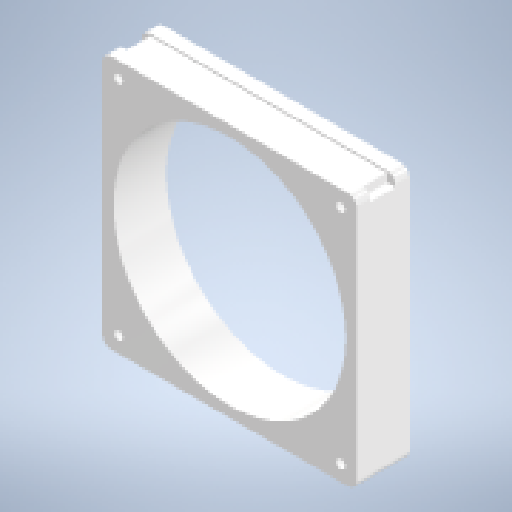
# Autodesk Inventor part: Body
Saved by Autodesk Inventor 2023.1 (Build 271208000, 208)
## iProperties
Created: 2023-11-19
Part Number: Body
Material: ABS Plastic
Document SubType Name: Modeling
Designer: Vinicius
Density: 1.06 g/cm^3
Appearance: Rubber - Black
Author: Vinicius
Autodesk Inventor part; units mm, degrees
ref_plane "YZ Plane" through (0, 0, 0) normal (1, 0, 0) x (0, 1, 0)
ref_plane "XZ Plane" through (0, 0, 0) normal (0, 1, 0) x (-1, 0, 0)
ref_plane "XY Plane" through (0, 0, 0) normal (0, 0, 1) x (1, 0, 0)
sketch "Sketch1" plane through (0, 0, 0) normal (0, 0, 1) x (1, 0, 0)
  line L0 (-56, 60) -> (56, 60)
  line L1 (60, 56) -> (60, -56)
  line L2 (56, -60) -> (-56, -60)
  line L3 (-60, -56) -> (-60, 56)
  line L4 (-60, 60) -> (60, -60) construction
  line L5 (60, 60) -> (-60, -60) construction
  circle A0 centre (0, 0) radius 55
  line L6 (-52.5, 52.5) -> (52.5, 52.5) construction
  line L7 (52.5, 52.5) -> (52.5, -52.5) construction
  line L8 (52.5, -52.5) -> (-52.5, -52.5) construction
  line L9 (-52.5, -52.5) -> (-52.5, 52.5) construction
  line L10 (-52.5, 52.5) -> (52.5, -52.5) construction
  line L11 (52.5, 52.5) -> (-52.5, -52.5) construction
  circle A1 centre (-52.5, 52.5) radius 2.15
  circle A2 centre (-52.5, -52.5) radius 2.15
  circle A3 centre (52.5, -52.5) radius 2.15
  circle A4 centre (52.5, 52.5) radius 2.15
  arc A5 (-56, 60) -> (-60, 56) centre (-56, 56) ccw
  arc A6 (-60, -56) -> (-56, -60) centre (-56, -56) ccw
  arc A7 (56, -60) -> (60, -56) centre (56, -56) ccw
  arc A8 (60, 56) -> (56, 60) centre (56, 56) ccw
  dimension "d0" = 120
  dimension "d1" = 120
  dimension "d2" = 110
  dimension "d3" = 105
  dimension "d4" = 4.3
  dimension "d5" = 4.3
  dimension "d6" = 4.3
  dimension "d7" = 4.3
  dimension "d8" = 4
  constraints: 24 end point, 9 centre point, 8 point on circle, 8 point on line, 8 tangent, 4 coincident, 4 midpoint, 4 parallel, 3 equal radius, 3 perpendicular, 2 horizontal
  measures "d0" distance of L4.end L5.end
  measures "d1" distance of L5.start L4.end
  measures "d2" diameter of A0
  measures "d3" distance of L7.end L8.end
  measures "d4" diameter of A1
  measures "d5" diameter of A2
  measures "d6" diameter of A3
  measures "d7" diameter of A4
  measures "d8" radius of A5
extrude "Extrusion1" add sketch "Sketch1" along normal mid plane 25
sketch "Sketch3" plane through (-56, 60, -12.5) normal (0, 1, 0) x (1, 0, 0)
  line L0 (-4, -5.5) -> (116, -5.5)
  line L1 (116, -5.5) -> (116, -19.5)
  line L2 (116, -19.5) -> (-4, -19.5)
  line L3 (-4, -19.5) -> (-4, -5.5)
  line L4 (-4, -5.5) -> (116, -19.5) construction
  line L5 (116, -5.5) -> (-4, -19.5) construction
  line L6 (-4, 0) -> (-4, -25) projected
  line L7 (116, 0) -> (116, -25) projected
  point P0 (56, -12.5)
  point P1 (-4, -12.5)
  dimension "d15" = 14
  constraints: 12 end point, 4 midpoint, 2 parallel, 1 horizontal, 1 perpendicular
  measures "d15" distance between parallel lines of L2 L0
extrude "Extrusion3" cut sketch "Sketch3" against normal blind 0.9
sketch "Sketch4" plane through (-56, 59.1, -12.5) normal (0, 1, 0) x (1, 0, 0)
  line L0 (114.5278, -5.5) -> (114.5278, -19.5) projected
  line L1 (-2.5278, -5.5) -> (114.5278, -5.5) projected
  line L2 (-2.5278, -19.5) -> (-2.5278, -5.5) projected
  line L3 (114.5278, -19.5) -> (-2.5278, -19.5) projected
  line L4 (116, 0) -> (116, -25) projected
  line L5 (-4, 0) -> (-4, -25) projected
  line L6 (116, 0) -> (116, -25) projected
  line L7 (114.5278, -19.5) -> (-2.5278, -19.5) projected
  line L8 (116, -5.5) -> (112, -5.5)
  line L9 (112, -5.5) -> (112, -19.5)
  line L10 (112, -19.5) -> (116, -19.5)
  line L11 (116, -19.5) -> (116, -5.5)
  line L12 (-4, -5.5) -> (0, -5.5)
  line L13 (0, -5.5) -> (0, -19.5)
  line L14 (0, -19.5) -> (-4, -19.5)
  line L15 (-4, -19.5) -> (-4, -5.5)
  point P0 (56, -12.5)
  point P1 (116, -19.5)
  point P2 (116, -5.5)
  point P3 (-4, -19.5)
  point P4 (-2.5278, -19.5)
  dimension "d18" = 4
  dimension "d19" = 4
  constraints: 16 end point, 6 point on line, 4 parallel, 2 horizontal, 2 perpendicular
  measures "d18" distance from line of L9 L8.start
  measures "d19" distance between parallel lines of L15 L13
extrude "Extrusion4" cut sketch "Sketch4" against normal blind 4 contours L8 L4 L10 L0 | L0 L3 L9 L1 | L13 L3 L2 L1 | L2 L14 L5 L12
equation "\"d0\" = Size"
equation "\"d1\" = Size"
equation "\"d2\" = DuctDiammeter"
equation "\"d3\" = DistanceBetweenHoles"
equation "\"d8\" = CornerRadius"
equation "\"d9\" = Depth"
equation "\"Size\" = 120"
equation "\"DistanceBetweenHoles\" = 105"
equation "\"DuctDiammeter\" = 110"
equation "\"CornerRadius\" = 4"
equation "\"Depth\" = 25"
body "Solid1"
